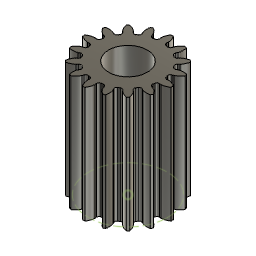
Assembly v3 (Autodesk Fusion 360 archive; units mm, degrees)
design "GEARS_Spur Gear (16 teeth)"
description: Spur Gear; Module: 0.637; Num Teeth: 16; Pressure Angle: 20.0; Backlash: 0.20 mm
Autodesk Fusion 360 part; units mm, degrees
sketch "Sketch1" plane through (0, 0, 0) normal (0, 0, 1) x (1, 0, 0)
  circle A0 centre (0, 0) radius 4.2808
  circle A1 centre (0, 0) radius 2.5
extrude "Extrude1" add sketch "Sketch1" along normal blind 10
sketch "Sketch2" plane through (0, 0, 0) normal (0, 0, 1) x (1, 0, 0)
  spline S0 degree 5 poles (4.7632, -0.4936) (4.7659, -0.4939) (4.7714, -0.4944) (4.7796, -0.4949) (4.7906, -0.4951) (4.8044, -0.4948) (4.8181, -0.494) (4.832, -0.493) (4.8458, -0.4918) (4.8596, -0.4905) (4.8735, -0.4891) (4.8874, -0.4875) (4.9013, -0.4858) (4.9151, -0.4839) (4.929, -0.4817) (4.943, -0.4794) (4.9569, -0.4768) (4.9708, -0.4741) (4.9847, -0.4713) (4.9986, -0.4684) (5.0126, -0.4653) (5.0265, -0.4622) (5.0404, -0.4589) (5.0544, -0.4554) (5.0683, -0.4518) (5.0823, -0.4481) (5.0962, -0.4443) (5.1101, -0.4403) (5.1241, -0.4362) (5.138, -0.432) (5.152, -0.4277) (5.1659, -0.4233) (5.1798, -0.4188) (5.1938, -0.4141) (5.2077, -0.4094) (5.2216, -0.4045) (5.2355, -0.3995) (5.2494, -0.3945) (5.2634, -0.3893) (5.2773, -0.384) (5.2912, -0.3786) (5.305, -0.3731) (5.3189, -0.3675) (5.3328, -0.3618) (5.3467, -0.356) (5.3605, -0.3501) (5.3744, -0.3441) (5.3883, -0.338) (5.4021, -0.3318) (5.4159, -0.3256) (5.4298, -0.3192) (5.4436, -0.3127) (5.4574, -0.3061) (5.4712, -0.2995) (5.4849, -0.2927) (5.4987, -0.2859) (5.5125, -0.2789) (5.5262, -0.2719) (5.54, -0.2648) (5.5537, -0.2576) (5.5674, -0.2503) (5.5811, -0.2429) (5.5948, -0.2354) (5.6085, -0.2278) (5.6221, -0.2202) (5.6358, -0.2124) (5.6494, -0.2046) (5.663, -0.1967) (5.6766, -0.1887) (5.6902, -0.1806) (5.7038, -0.1724) (5.7146, -0.1658) (5.7228, -0.1608) (5.7282, -0.1574) (5.7309, -0.1558) knots 0 0 0 0 0 0 0.01428571 0.02857143 0.04285714 0.05714286 0.07142857 0.08571429 0.1 0.11428571 0.12857143 0.14285714 0.15714286 0.17142857 0.18571429 0.2 0.21428571 0.22857143 0.24285714 0.25714286 0.27142857 0.28571429 0.3 0.31428571 0.32857143 0.34285714 0.35714286 0.37142857 0.38571429 0.4 0.41428571 0.42857143 0.44285714 0.45714286 0.47142857 0.48571429 0.5 0.51428571 0.52857143 0.54285714 0.55714286 0.57142857 0.58571429 0.6 0.61428571 0.62857143 0.64285714 0.65714286 0.67142857 0.68571429 0.7 0.71428571 0.72857143 0.74285714 0.75714286 0.77142857 0.78571429 0.8 0.81428571 0.82857143 0.84285714 0.85714286 0.87142857 0.88571429 0.9 0.91428571 0.92857143 0.94285714 0.95714286 0.97142857 0.98571429 1 1 1 1 1 1
  spline S1 degree 5 poles (4.7632, 0.4936) (4.7659, 0.4939) (4.7714, 0.4944) (4.7796, 0.4949) (4.7906, 0.4951) (4.8044, 0.4948) (4.8181, 0.494) (4.832, 0.493) (4.8458, 0.4918) (4.8596, 0.4905) (4.8735, 0.4891) (4.8874, 0.4875) (4.9013, 0.4858) (4.9151, 0.4839) (4.929, 0.4817) (4.943, 0.4794) (4.9569, 0.4768) (4.9708, 0.4741) (4.9847, 0.4713) (4.9986, 0.4684) (5.0126, 0.4653) (5.0265, 0.4622) (5.0404, 0.4589) (5.0544, 0.4554) (5.0683, 0.4518) (5.0823, 0.4481) (5.0962, 0.4443) (5.1101, 0.4403) (5.1241, 0.4362) (5.138, 0.432) (5.152, 0.4277) (5.1659, 0.4233) (5.1798, 0.4188) (5.1938, 0.4141) (5.2077, 0.4094) (5.2216, 0.4045) (5.2355, 0.3995) (5.2494, 0.3945) (5.2634, 0.3893) (5.2773, 0.384) (5.2912, 0.3786) (5.305, 0.3731) (5.3189, 0.3675) (5.3328, 0.3618) (5.3467, 0.356) (5.3605, 0.3501) (5.3744, 0.3441) (5.3883, 0.338) (5.4021, 0.3318) (5.4159, 0.3256) (5.4298, 0.3192) (5.4436, 0.3127) (5.4574, 0.3061) (5.4712, 0.2995) (5.4849, 0.2927) (5.4987, 0.2859) (5.5125, 0.2789) (5.5262, 0.2719) (5.54, 0.2648) (5.5537, 0.2576) (5.5674, 0.2503) (5.5811, 0.2429) (5.5948, 0.2354) (5.6085, 0.2278) (5.6221, 0.2202) (5.6358, 0.2124) (5.6494, 0.2046) (5.663, 0.1967) (5.6766, 0.1887) (5.6902, 0.1806) (5.7038, 0.1724) (5.7146, 0.1658) (5.7228, 0.1608) (5.7282, 0.1574) (5.7309, 0.1558) knots 0 0 0 0 0 0 0.01428571 0.02857143 0.04285714 0.05714286 0.07142857 0.08571429 0.1 0.11428571 0.12857143 0.14285714 0.15714286 0.17142857 0.18571429 0.2 0.21428571 0.22857143 0.24285714 0.25714286 0.27142857 0.28571429 0.3 0.31428571 0.32857143 0.34285714 0.35714286 0.37142857 0.38571429 0.4 0.41428571 0.42857143 0.44285714 0.45714286 0.47142857 0.48571429 0.5 0.51428571 0.52857143 0.54285714 0.55714286 0.57142857 0.58571429 0.6 0.61428571 0.62857143 0.64285714 0.65714286 0.67142857 0.68571429 0.7 0.71428571 0.72857143 0.74285714 0.75714286 0.77142857 0.78571429 0.8 0.81428571 0.82857143 0.84285714 0.85714286 0.87142857 0.88571429 0.9 0.91428571 0.92857143 0.94285714 0.95714286 0.97142857 0.98571429 1 1 1 1 1 1
  arc A0 (5.7309, -0.1558) -> (5.7309, 0.1558) centre (0, 0) ccw
  line L0 (4.248, -0.4413) -> (4.7632, -0.4936)
  line L1 (4.248, 0.4413) -> (4.7632, 0.4936)
  line L2 (4.248, -0.4413) -> (4.248, 0.4413)
  point P0 (4.831, -0.493)
  point P1 (4.8995, -0.486)
  point P2 (4.9684, -0.4746)
  point P3 (5.0376, -0.4595)
  point P4 (5.1069, -0.4412)
  point P5 (5.1764, -0.4199)
  point P6 (5.2459, -0.3957)
  point P7 (5.3155, -0.3689)
  point P8 (5.3851, -0.3394)
  point P9 (5.4545, -0.3075)
  point P10 (5.5239, -0.2731)
  point P11 (5.5931, -0.2363)
  point P12 (5.6621, -0.1972)
  point P13 (4.831, 0.493)
  point P14 (4.8995, 0.486)
  point P15 (4.9684, 0.4746)
  point P16 (5.0376, 0.4595)
  point P17 (5.1069, 0.4412)
  point P18 (5.1764, 0.4199)
  point P19 (5.2459, 0.3957)
  point P20 (5.3155, 0.3689)
  point P21 (5.3851, 0.3394)
  point P22 (5.4545, 0.3075)
  point P23 (5.5239, 0.2731)
  point P24 (5.5931, 0.2363)
  point P25 (5.6621, 0.1972)
extrude "Extrude2" add sketch "Sketch2" along normal blind 10
fillet "Fillet1" radius 0.3 2 edges at (4.2579, -0.4423, 5) (4.2579, 0.4423, 5)
pattern_circular "C-Pattern1" count 16 over 360 about axis through (0, 0, 0) along (0, 0, 1) of "Extrude2", "Fillet1"
sketch "Sketch3" plane through (0, 0, 0) normal (0, 0, 1) x (1, 0, 0)
  circle A0 centre (0, 0) radius 5.096 construction
extrude "Extrude3" add 1 faces at (3.6763, 0, 10) along direction (0, 0, 1) blind 5
